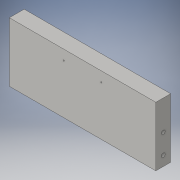
# Autodesk Inventor part: SideWall
Saved by Autodesk Inventor 2016 (Build 200138000, 138)
## iProperties
Created: 2017-01-04
Part Number: SideWall
Material: Generic
Document SubType Name: Modeling
Designer: james
Density: 1 g/cm^3
Appearance: Default
Author: james
Autodesk Inventor part; units mm, degrees
ref_plane "YZ Plane" through (0, 0, 0) normal (1, 0, 0) x (0, 1, 0)
ref_plane "XZ Plane" through (0, 0, 0) normal (0, 1, 0) x (-1, 0, 0)
ref_plane "XY Plane" through (0, 0, 0) normal (0, 0, 1) x (1, 0, 0)
sketch "Sketch1" plane through (0, 0, 0) normal (0, 1, 0) x (-1, 0, 0)
  line L0 (75.3001, 36.8452) -> (-112.6599, 36.8452)
  line L1 (-112.6599, 36.8452) -> (-112.6599, 17.7952)
  line L2 (-112.6599, 17.7952) -> (75.3001, 17.7952)
  line L3 (75.3001, 17.7952) -> (75.3001, 36.8452)
  point P0 (0, 0)
  dimension "d0" = 187.96
  dimension "d1" = 19.05
  constraints: 8 end point, 2 parallel, 1 horizontal, 1 perpendicular
  measures "d0" distance of L1.end L2.end
  measures "d1" distance of L2.end L0.start
extrude "Extrusion1" add sketch "Sketch1" along normal blind 76.2
sketch "Sketch2" plane through (112.6599, 0, 36.8452) normal (1, 0, 0) x (0, 0, -1)
  line L0 (0, 0) -> (0, 76.2) projected
  line L1 (0, 0) -> (19.05, 0) projected
  point P0 (36.8452, 0)
  point P1 (9.525, 12.7)
  point P2 (9.525, 38.1)
  dimension "d4" = 0
  dimension "d5" = 9.525
  dimension "d6" = 25.4
  dimension "d7" = 12.7
  measures "d4" horizontal distance of point (9.525, 12.7) point (9.525, 38.1)
  measures "d5" distance from line of L0 point (9.525, 38.1)
  measures "d6" distance of point (9.525, 12.7) point (9.525, 38.1)
  measures "d7" distance from line of L1 point (9.525, 12.7)
hole "Hole1" at (112.6599, 12.7, 27.3202) at (112.6599, 38.1, 27.3202) direction (-1, 0, 0) diameter 4.9149 end through all
sketch "Sketch4" plane through (112.6599, 0, 17.7952) normal (0, 0, -1) x (-1, 0, 0)
  line L0 (19.05, 57.15) -> (168.91, 57.15)
  line L1 (168.91, 57.15) -> (168.91, 12.7)
  line L2 (168.91, 12.7) -> (19.05, 12.7)
  line L3 (19.05, 12.7) -> (19.05, 57.15)
  line L4 (0, 76.2) -> (187.96, 76.2) projected
  line L5 (0, 0) -> (187.96, 0) projected
  point P0 (112.6599, 0)
  dimension "d21" = 19.05
  dimension "d22" = 12.7
  dimension "d23" = 19.05
  dimension "d24" = 19.05
  constraints: 8 end point, 2 parallel, 1 horizontal, 1 perpendicular
  measures "d21" distance between parallel lines of L0 L4
  measures "d22" distance between parallel lines of L2 L5
  measures "d23" horizontal distance of L5.end L1.end
  measures "d24" horizontal distance of L5.start L2.end
extrude "Extrusion3" cut sketch "Sketch4" against normal blind 5.08
sketch "Sketch5" plane through (112.6599, 0, 17.7952) normal (0, 0, -1) x (-1, 0, 0)
  line L0 (187.96, 0) -> (187.96, 76.2) projected
  line L1 (0, 0) -> (0, 76.2) projected
  line L2 (0, 76.2) -> (187.96, 76.2) projected
  point P0 (112.6599, 0)
  point P1 (69.85, 63.5)
  point P2 (118.11, 63.5)
  dimension "d27" = 48.26
  dimension "d28" = 69.85
  dimension "d30" = 12.7
  dimension "d31" = 12.7
  dimension "d32" = 69.85
  measures "d27" distance of point (69.85, 63.5) point (118.11, 63.5)
  measures "d28" distance from line of L0 point (118.11, 63.5)
  measures "d30" distance from line of point (69.85, 63.5) L2
  measures "d31" distance from line of point (118.11, 63.5) L2
  measures "d32" horizontal distance of point (69.85, 63.5) L1.end
hole "Hole2" at (42.8099, 63.5, 17.7952) at (-5.4501, 63.5, 17.7952) direction (0, 0, 1) diameter 1.524 end through all
sketch "Sketch6" plane through (112.6599, 0, 22.8752) normal (0, 0, -1) x (-1, 0, 0)
  line L0 (25.8304, 53.7302) -> (132.9321, 53.7302) construction
  line L1 (132.9321, 53.7302) -> (132.9321, 26.2821) construction
  line L2 (132.9321, 26.2821) -> (25.8304, 26.2821) construction
  line L3 (25.8304, 26.2821) -> (25.8304, 53.7302) construction
  line L4 (34.7951, 51.1546) -> (34.7951, 41.0658)
  line L5 (34.7951, 41.0658) -> (36.5312, 41.0658)
  spline S0 degree 2 poles (36.5312, 41.0658) (37.4988, 41.0658) (38.2957, 40.3543) (38.2957, 39.7709) knots 0 0 0 1 2 2 2
  spline S1 degree 2 poles (38.2957, 39.7709) (38.2957, 39.1875) (37.4988, 38.4902) (36.5312, 38.4902) knots 0 0 0 1 2 2 2
  line L6 (36.5312, 38.4902) -> (30.4978, 38.4902)
  spline S2 degree 2 poles (30.4978, 38.4902) (29.5302, 38.4902) (28.7333, 39.2017) (28.7333, 39.7851) knots 0 0 0 1 2 2 2
  spline S3 degree 2 poles (28.7333, 39.7851) (28.7333, 40.3685) (29.5302, 41.0658) (30.4978, 41.0658) knots 0 0 0 1 2 2 2
  line L7 (30.4978, 41.0658) -> (32.2196, 41.0658)
  line L8 (32.2196, 41.0658) -> (32.2196, 51.1546)
  line L9 (32.2196, 51.1546) -> (29.4306, 51.1546)
  line L10 (29.4306, 51.1546) -> (29.4306, 48.7214)
  spline S4 degree 2 poles (29.4306, 48.7214) (29.4306, 47.7537) (28.7191, 46.9569) (28.1357, 46.9569) knots 0 0 0 1 2 2 2
  spline S5 degree 2 poles (28.1357, 46.9569) (27.5522, 46.9569) (26.855, 47.7537) (26.855, 48.7214) knots 0 0 0 1 2 2 2
  line L11 (26.855, 48.7214) -> (26.855, 53.7302)
  line L12 (26.855, 53.7302) -> (40.2024, 53.7302)
  line L13 (40.2024, 53.7302) -> (40.2024, 48.7214)
  spline S6 degree 2 poles (40.2024, 48.7214) (40.2024, 47.7537) (39.4909, 46.9569) (38.9075, 46.9569) knots 0 0 0 1 2 2 2
  spline S7 degree 2 poles (38.9075, 46.9569) (38.3241, 46.9569) (37.6269, 47.7537) (37.6269, 48.7214) knots 0 0 0 1 2 2 2
  line L14 (37.6269, 48.7214) -> (37.6269, 51.1546)
  line L15 (37.6269, 51.1546) -> (34.7951, 51.1546)
  line L16 (55.4567, 42.8872) -> (44.884, 42.8872)
  spline S8 degree 2 poles (44.884, 42.8872) (45.2824, 41.8769) (47.3315, 40.6531) (49.0818, 40.6531) knots 0 0 0 1 2 2 2
  spline S9 degree 2 poles (49.0818, 40.6531) (50.519, 40.6531) (52.8953, 41.265) knots 0 0 0 1 1 1
  spline S10 degree 2 poles (52.8953, 41.265) (53.8772, 41.5211) (54.2471, 41.5211) knots 0 0 0 1 1 1
  spline S11 degree 2 poles (54.2471, 41.5211) (54.7736, 41.5211) (55.4709, 40.7954) (55.4709, 40.2405) knots 0 0 0 1 2 2 2
  spline S12 degree 2 poles (55.4709, 40.2405) (55.4709, 39.7424) (55.1009, 39.3867) knots 0 0 0 1 1 1
  spline S13 degree 2 poles (55.1009, 39.3867) (54.5887, 38.9171) (50.6897, 38.0776) (48.8968, 38.0776) knots 0 0 0 1 2 2 2
  spline S14 degree 2 poles (48.8968, 38.0776) (45.8089, 38.0776) (42.095, 41.5638) (42.095, 44.1109) knots 0 0 0 1 2 2 2
  spline S15 degree 2 poles (42.095, 44.1109) (42.095, 46.8288) (46.1078, 50.2297) (48.726, 50.2297) knots 0 0 0 1 2 2 2
  spline S16 degree 2 poles (48.726, 50.2297) (50.2913, 50.2297) (52.9238, 49.1198) (53.5641, 48.4795) knots 0 0 0 1 2 2 2
  spline S17 degree 2 poles (53.5641, 48.4795) (54.4606, 47.5545) (55.0582, 46.1885) knots 0 0 0 1 1 1
  spline S18 degree 2 poles (55.0582, 46.1885) (55.4567, 45.2351) (55.4567, 43.9829) knots 0 0 0 1 1 1
  line L17 (55.4567, 43.9829) -> (55.4567, 42.8872)
  spline S19 degree 2 poles (52.6107, 45.4628) (52.0131, 46.5584) (50.1063, 47.6541) (48.7829, 47.6541) knots 0 0 0 1 2 2 2
  spline S20 degree 2 poles (48.7829, 47.6541) (47.4738, 47.6541) (45.5528, 46.5584) (44.9551, 45.4628) knots 0 0 0 1 2 2 2
  line L18 (44.9551, 45.4628) -> (52.6107, 45.4628)
  line L19 (66.7408, 38.4902) -> (66.7408, 39.0879)
  spline S21 degree 2 poles (66.7408, 39.0879) (65.7732, 38.5898) (63.4395, 38.0776) (62.4861, 38.0776) knots 0 0 0 1 2 2 2
  spline S22 degree 2 poles (62.4861, 38.0776) (60.4228, 38.0776) (57.833, 40.2689) (57.833, 41.5923) knots 0 0 0 1 2 2 2
  spline S23 degree 2 poles (57.833, 41.5923) (57.833, 43.2145) (61.1343, 45.975) (64.0372, 45.975) knots 0 0 0 1 2 2 2
  spline S24 degree 2 poles (64.0372, 45.975) (65.204, 45.975) (66.7408, 45.7189) knots 0 0 0 1 1 1
  line L20 (66.7408, 45.7189) -> (66.7408, 46.345)
  spline S25 degree 2 poles (66.7408, 46.345) (66.7408, 46.9284) (65.7447, 47.6541) (64.3644, 47.6541) knots 0 0 0 1 2 2 2
  spline S26 degree 2 poles (64.3644, 47.6541) (63.2118, 47.6541) (61.3904, 47.1988) knots 0 0 0 1 1 1
  spline S27 degree 2 poles (61.3904, 47.1988) (60.7216, 47.0423) (60.3374, 47.0423) knots 0 0 0 1 1 1
  spline S28 degree 2 poles (60.3374, 47.0423) (59.8252, 47.0423) (59.1137, 47.7822) (59.1137, 48.3656) knots 0 0 0 1 2 2 2
  spline S29 degree 2 poles (59.1137, 48.3656) (59.1137, 48.6929) (59.3698, 49.1625) (59.8109, 49.4471) (60.5367, 49.6463) knots 0 0 0 1 2 3 3 3
  spline S30 degree 2 poles (60.5367, 49.6463) (61.4901, 49.9167) (63.468, 50.2297) (64.2648, 50.2297) knots 0 0 0 1 2 2 2
  spline S31 degree 2 poles (64.2648, 50.2297) (66.6697, 50.2297) (69.3164, 48.1522) (69.3164, 46.3592) knots 0 0 0 1 2 2 2
  line L21 (69.3164, 46.3592) -> (69.3164, 41.0658)
  line L22 (69.3164, 41.0658) -> (69.7575, 41.0658)
  spline S32 degree 2 poles (69.7575, 41.0658) (70.7251, 41.0658) (71.522, 40.3543) (71.522, 39.7709) knots 0 0 0 1 2 2 2
  spline S33 degree 2 poles (71.522, 39.7709) (71.522, 39.1875) (70.7251, 38.4902) (69.7575, 38.4902) knots 0 0 0 1 2 2 2
  line L23 (69.7575, 38.4902) -> (66.7408, 38.4902)
  spline S34 degree 2 poles (66.7408, 43.1006) (65.204, 43.3995) (63.8949, 43.3995) knots 0 0 0 1 1 1
  spline S35 degree 2 poles (63.8949, 43.3995) (62.3296, 43.3995) (61.1912, 42.6311) knots 0 0 0 1 1 1
  spline S36 degree 2 poles (61.1912, 42.6311) (60.494, 42.1472) (60.494, 41.6492) knots 0 0 0 1 1 1
  spline S37 degree 2 poles (60.494, 41.6492) (60.494, 41.2935) (60.8355, 41.0658) knots 0 0 0 1 1 1
  spline S38 degree 2 poles (60.8355, 41.0658) (61.4616, 40.6531) (62.5573, 40.6531) knots 0 0 0 1 1 1
  spline S39 degree 2 poles (62.5573, 40.6531) (63.4822, 40.6531) (65.8301, 41.3788) (66.7408, 42.0049) knots 0 0 0 1 2 2 2
  line L24 (66.7408, 42.0049) -> (66.7408, 43.1006)
  line L25 (75.8905, 49.9024) -> (75.8905, 49.1767)
  spline S40 degree 2 poles (75.8905, 49.1767) (76.5166, 49.7886) (77.5411, 50.2439) (78.2099, 50.2439) knots 0 0 0 1 2 2 2
  spline S41 degree 2 poles (78.2099, 50.2439) (78.7649, 50.2439) (79.8748, 49.689) (80.4013, 49.1483) knots 0 0 0 1 2 2 2
  spline S42 degree 2 poles (80.4013, 49.1483) (81.0701, 49.689) (82.4362, 50.2297) (83.1619, 50.2297) knots 0 0 0 1 2 2 2
  spline S43 degree 2 poles (83.1619, 50.2297) (84.5848, 50.2297) (85.4813, 49.4613) knots 0 0 0 1 1 1
  spline S44 degree 2 poles (85.4813, 49.4613) (86.6624, 48.4652) (86.6624, 46.8288) knots 0 0 0 1 1 1
  line L26 (86.6624, 46.8288) -> (86.6624, 41.0658)
  spline S45 degree 2 poles (86.6624, 41.0658) (87.63, 41.0658) (88.4269, 40.3543) (88.4269, 39.7709) knots 0 0 0 1 2 2 2
  spline S46 degree 2 poles (88.4269, 39.7709) (88.4269, 39.1875) (87.63, 38.4902) (86.6624, 38.4902) knots 0 0 0 1 2 2 2
  line L27 (86.6624, 38.4902) -> (84.0868, 38.4902)
  line L28 (84.0868, 38.4902) -> (84.0868, 46.6154)
  spline S47 degree 2 poles (84.0868, 46.6154) (84.0868, 47.1988) (83.6599, 47.6541) (83.2188, 47.6541) knots 0 0 0 1 2 2 2
  spline S48 degree 2 poles (83.2188, 47.6541) (82.7919, 47.6541) (82.4219, 47.4265) knots 0 0 0 1 1 1
  spline S49 degree 2 poles (82.4219, 47.4265) (81.9666, 47.1134) (81.2978, 46.2596) knots 0 0 0 1 1 1
  line L29 (81.2978, 46.2596) -> (81.2978, 41.0658)
  spline S50 degree 2 poles (81.2978, 41.0658) (82.2654, 41.0658) (83.0623, 40.3543) (83.0623, 39.7709) knots 0 0 0 1 2 2 2
  spline S51 degree 2 poles (83.0623, 39.7709) (83.0623, 39.1875) (82.2654, 38.4902) (81.2978, 38.4902) knots 0 0 0 1 2 2 2
  line L30 (81.2978, 38.4902) -> (78.7222, 38.4902)
  line L31 (78.7222, 38.4902) -> (78.7222, 46.6296)
  spline S52 degree 2 poles (78.7222, 46.6296) (78.7222, 47.1988) (78.2811, 47.6684) (77.84, 47.6684) knots 0 0 0 1 2 2 2
  spline S53 degree 2 poles (77.84, 47.6684) (77.3846, 47.6684) (76.5024, 47.0992) (75.8905, 46.2596) knots 0 0 0 1 2 2 2
  line L32 (75.8905, 46.2596) -> (75.8905, 41.0658)
  spline S54 degree 2 poles (75.8905, 41.0658) (76.8581, 41.0658) (77.655, 40.3543) (77.655, 39.7709) knots 0 0 0 1 2 2 2
  spline S55 degree 2 poles (77.655, 39.7709) (77.655, 39.1875) (76.8581, 38.4902) (75.8905, 38.4902) knots 0 0 0 1 2 2 2
  line L33 (75.8905, 38.4902) -> (73.3149, 38.4902)
  spline S56 degree 2 poles (73.3149, 38.4902) (72.3473, 38.4902) (71.5504, 39.2017) (71.5504, 39.7851) knots 0 0 0 1 2 2 2
  spline S57 degree 2 poles (71.5504, 39.7851) (71.5504, 40.3685) (72.3473, 41.0658) (73.3149, 41.0658) knots 0 0 0 1 2 2 2
  line L34 (73.3149, 41.0658) -> (73.3149, 47.3269)
  spline S58 degree 2 poles (73.3149, 47.3269) (72.3473, 47.3269) (71.5504, 48.0383) (71.5504, 48.6218) knots 0 0 0 1 2 2 2
  spline S59 degree 2 poles (71.5504, 48.6218) (71.5504, 49.2052) (72.3473, 49.9024) (73.3149, 49.9024) knots 0 0 0 1 2 2 2
  line L35 (73.3149, 49.9024) -> (75.8905, 49.9024)
  point P0 (112.6599, 0)
  constraints: 2 other
extrude "Extrusion4" add sketch "Sketch6" along normal blind 2.54
sketch "Sketch7" plane through (112.6599, 0, 22.8752) normal (0, 0, -1) x (-1, 0, 0)
  line L0 (44.6427, 45.8411) -> (161.4517, 31.4988) construction
  line L1 (161.4517, 31.4988) -> (158.1503, 4.6114) construction
  line L2 (158.1503, 4.6114) -> (41.3413, 18.9537) construction
  line L3 (41.3413, 18.9537) -> (44.6427, 45.8411) construction
  line L4 (48.3943, 34.8288) -> (47.9989, 31.6086)
  line L5 (47.9989, 31.6086) -> (48.917, 31.4959)
  spline S0 degree 2 poles (48.917, 31.4959) (49.8774, 31.3779) (50.5816, 30.5747) (50.5105, 29.9956) knots 0 0 0 1 2 2 2
  spline S1 degree 2 poles (50.5105, 29.9956) (50.4394, 29.4165) (49.5635, 28.8216) (48.6031, 28.9395) knots 0 0 0 1 2 2 2
  line L6 (48.6031, 28.9395) -> (44.7332, 29.4147)
  spline S2 degree 2 poles (44.7332, 29.4147) (43.7728, 29.5326) (43.0686, 30.3359) (43.1397, 30.9149) knots 0 0 0 1 2 2 2
  spline S3 degree 2 poles (43.1397, 30.9149) (43.2108, 31.494) (44.0867, 32.089) (45.0471, 31.971) knots 0 0 0 1 2 2 2
  line L7 (45.0471, 31.971) -> (45.4426, 31.9225)
  line L8 (45.4426, 31.9225) -> (46.6721, 41.9361)
  line L9 (46.6721, 41.9361) -> (46.2766, 41.9847)
  spline S4 degree 2 poles (46.2766, 41.9847) (45.3162, 42.1026) (44.612, 42.9059) (44.6831, 43.485) knots 0 0 0 1 2 2 2
  spline S5 degree 2 poles (44.6831, 43.485) (44.7525, 44.0499) (45.6301, 44.659) (46.5905, 44.5411) knots 0 0 0 1 2 2 2
  line L10 (46.5905, 44.5411) -> (52.3795, 43.8159)
  spline S6 degree 2 poles (52.3795, 43.8159) (55.0771, 43.4847) (57.7277, 40.4353) (57.4918, 38.5145) knots 0 0 0 1 2 2 2
  spline S7 degree 2 poles (57.4918, 38.5145) (57.3462, 37.3281) (55.7069, 35.5366) (54.2009, 34.9473) knots 0 0 0 1 2 2 2
  spline S8 degree 2 poles (54.2009, 34.9473) (54.9333, 34.1406) (55.7144, 32.9121) knots 0 0 0 1 1 1
  spline S9 degree 2 poles (55.7144, 32.9121) (56.2067, 32.1348) (56.9957, 30.5039) knots 0 0 0 1 1 1
  spline S10 degree 2 poles (56.9957, 30.5039) (57.9561, 30.386) (58.2091, 30.1112) knots 0 0 0 1 1 1
  spline S11 degree 2 poles (58.2091, 30.1112) (58.6603, 29.5827) (58.5892, 29.0036) knots 0 0 0 1 1 1
  spline S12 degree 2 poles (58.5892, 29.0036) (58.5181, 28.4246) (57.6422, 27.8296) (56.6818, 27.9475) knots 0 0 0 1 2 2 2
  line L11 (56.6818, 27.9475) -> (55.3683, 28.1088)
  spline S13 degree 2 poles (55.3683, 28.1088) (52.8507, 33.2924) (50.9225, 34.5184) knots 0 0 0 1 1 1
  line L12 (50.9225, 34.5184) -> (48.3943, 34.8288)
  line L13 (48.7082, 37.3852) -> (50.6996, 37.1406)
  spline S14 degree 2 poles (50.6996, 37.1406) (51.8154, 37.0036) (52.7327, 37.2351) knots 0 0 0 1 1 1
  spline S15 degree 2 poles (52.7327, 37.2351) (53.9605, 37.5431) (54.8869, 38.4329) (54.9476, 38.9272) knots 0 0 0 1 2 2 2
  spline S16 degree 2 poles (54.9476, 38.9272) (55.036, 39.6475) (53.6474, 41.0653) (52.1503, 41.2491) knots 0 0 0 1 2 2 2
  line L14 (52.1503, 41.2491) -> (49.2285, 41.6222)
  line L15 (49.2285, 41.6222) -> (48.7082, 37.3852)
  line L16 (72.5983, 30.4232) -> (62.1044, 31.7117)
  spline S17 degree 2 poles (62.1044, 31.7117) (62.3768, 30.6604) (64.2614, 29.196) (65.9986, 28.9827) knots 0 0 0 1 2 2 2
  spline S18 degree 2 poles (65.9986, 28.9827) (67.4251, 28.8076) (69.8583, 29.1253) knots 0 0 0 1 1 1
  spline S19 degree 2 poles (69.8583, 29.1253) (70.8641, 29.2599) (71.2313, 29.2148) knots 0 0 0 1 1 1
  spline S20 degree 2 poles (71.2313, 29.2148) (71.7539, 29.1506) (72.3575, 28.3453) (72.2899, 27.7945) knots 0 0 0 1 2 2 2
  spline S21 degree 2 poles (72.2899, 27.7945) (72.2292, 27.3002) (71.8186, 26.9922) knots 0 0 0 1 1 1
  spline S22 degree 2 poles (71.8186, 26.9922) (71.2529, 26.5885) (67.2807, 26.2304) (65.5012, 26.4489) knots 0 0 0 1 2 2 2
  spline S23 degree 2 poles (65.5012, 26.4489) (62.4363, 26.8252) (59.1749, 30.7381) (59.4853, 33.2663) knots 0 0 0 1 2 2 2
  spline S24 degree 2 poles (59.4853, 33.2663) (59.8166, 35.9639) (64.2139, 38.8504) (66.8126, 38.5313) knots 0 0 0 1 2 2 2
  spline S25 degree 2 poles (66.8126, 38.5313) (68.3662, 38.3405) (70.8439, 36.9181) (71.4014, 36.2045) knots 0 0 0 1 2 2 2
  spline S26 degree 2 poles (71.4014, 36.2045) (72.1784, 35.1772) (72.6052, 33.7485) knots 0 0 0 1 1 1
  spline S27 degree 2 poles (72.6052, 33.7485) (72.8844, 32.7536) (72.7318, 31.5108) knots 0 0 0 1 1 1
  line L17 (72.7318, 31.5108) -> (72.5983, 30.4232)
  spline S28 degree 2 poles (70.0875, 33.3265) (69.6278, 34.4868) (67.8688, 35.8067) (66.5553, 35.968) knots 0 0 0 1 2 2 2
  spline S29 degree 2 poles (66.5553, 35.968) (65.2559, 36.1275) (63.2157, 35.2741) (62.4889, 34.2594) knots 0 0 0 1 2 2 2
  line L18 (62.4889, 34.2594) -> (70.0875, 33.3265)
  line L19 (88.8072, 40.4184) -> (87.1355, 26.8032)
  line L20 (87.1355, 26.8032) -> (87.5733, 26.7495)
  spline S30 degree 2 poles (87.5733, 26.7495) (88.5337, 26.6315) (89.238, 25.8282) (89.1669, 25.2492) knots 0 0 0 1 2 2 2
  spline S31 degree 2 poles (89.1669, 25.2492) (89.0958, 24.6701) (88.2199, 24.0752) (87.2595, 24.1931) knots 0 0 0 1 2 2 2
  line L21 (87.2595, 24.1931) -> (84.2652, 24.5607)
  line L22 (84.2652, 24.5607) -> (84.3416, 25.1822)
  spline S32 degree 2 poles (84.3416, 25.1822) (83.4035, 24.7812) (81.4326, 24.4928) (80.4157, 24.6176) knots 0 0 0 1 2 2 2
  spline S33 degree 2 poles (80.4157, 24.6176) (77.5486, 24.9697) (74.4411, 28.7347) (74.7446, 31.2063) knots 0 0 0 1 2 2 2
  spline S34 degree 2 poles (74.7446, 31.2063) (75.0637, 33.805) (79.1991, 37.0104) (81.8543, 36.6844) knots 0 0 0 1 2 2 2
  spline S35 degree 2 poles (81.8543, 36.6844) (82.843, 36.563) (84.6892, 35.7199) (85.5451, 34.984) knots 0 0 0 1 2 2 2
  line L23 (85.5451, 34.984) -> (85.937, 38.1759)
  line L24 (85.937, 38.1759) -> (85.4992, 38.2297)
  spline S36 degree 2 poles (85.4992, 38.2297) (84.5387, 38.3476) (83.8328, 39.1368) (83.9039, 39.7158) knots 0 0 0 1 2 2 2
  spline S37 degree 2 poles (83.9039, 39.7158) (83.975, 40.2949) (84.8526, 40.904) (85.813, 40.786) knots 0 0 0 1 2 2 2
  line L25 (85.813, 40.786) -> (88.8072, 40.4184)
  spline S38 degree 2 poles (84.919, 29.8853) (85.1133, 31.4672) (83.1646, 33.9286) (81.5687, 34.1246) knots 0 0 0 1 2 2 2
  spline S39 degree 2 poles (81.5687, 34.1246) (79.9727, 34.3205) (77.4865, 32.4036) (77.2957, 30.85) knots 0 0 0 1 2 2 2
  spline S40 degree 2 poles (77.2957, 30.85) (77.1241, 29.4518) (78.8935, 27.3995) (80.7155, 27.1757) knots 0 0 0 1 2 2 2
  spline S41 degree 2 poles (80.7155, 27.1757) (82.5092, 26.9555) (84.7508, 28.5153) (84.919, 29.8853) knots 0 0 0 1 2 2 2
  line L26 (98.5866, 22.8023) -> (98.6594, 23.3955)
  spline S42 degree 2 poles (98.6594, 23.3955) (97.6383, 23.0191) (95.2596, 22.795) (94.3134, 22.9112) knots 0 0 0 1 2 2 2
  spline S43 degree 2 poles (94.3134, 22.9112) (92.2654, 23.1627) (89.962, 25.6533) (90.1233, 26.9668) knots 0 0 0 1 2 2 2
  spline S44 degree 2 poles (90.1233, 26.9668) (90.321, 28.5769) (93.9341, 30.9146) (96.8153, 30.5608) knots 0 0 0 1 2 2 2
  spline S45 degree 2 poles (96.8153, 30.5608) (97.9734, 30.4186) (99.4676, 29.9771) knots 0 0 0 1 1 1
  line L27 (99.4676, 29.9771) -> (99.5439, 30.5985)
  spline S46 degree 2 poles (99.5439, 30.5985) (99.615, 31.1776) (98.7148, 32.0193) (97.3448, 32.1875) knots 0 0 0 1 2 2 2
  spline S47 degree 2 poles (97.3448, 32.1875) (96.2007, 32.328) (94.3374, 32.098) knots 0 0 0 1 1 1
  spline S48 degree 2 poles (94.3374, 32.098) (93.6545, 32.0241) (93.2732, 32.071) knots 0 0 0 1 1 1
  spline S49 degree 2 poles (93.2732, 32.071) (92.7648, 32.1334) (92.1488, 32.9545) (92.2199, 33.5336) knots 0 0 0 1 2 2 2
  spline S50 degree 2 poles (92.2199, 33.5336) (92.2597, 33.8584) (92.5712, 34.2933) (93.0437, 34.522) (93.7883, 34.6313) knots 0 0 0 1 2 3 3 3
  spline S51 degree 2 poles (93.7883, 34.6313) (94.7675, 34.7835) (96.7689, 34.8531) (97.5598, 34.756) knots 0 0 0 1 2 2 2
  spline S52 degree 2 poles (97.5598, 34.756) (99.9467, 34.463) (102.3205, 32.0783) (102.102, 30.2988) knots 0 0 0 1 2 2 2
  line L28 (102.102, 30.2988) -> (101.4569, 25.0448)
  line L29 (101.4569, 25.0448) -> (101.8947, 24.991)
  spline S53 degree 2 poles (101.8947, 24.991) (102.8551, 24.8731) (103.5593, 24.0698) (103.4882, 23.4907) knots 0 0 0 1 2 2 2
  spline S54 degree 2 poles (103.4882, 23.4907) (103.4171, 22.9117) (102.5412, 22.3167) (101.5808, 22.4346) knots 0 0 0 1 2 2 2
  line L30 (101.5808, 22.4346) -> (98.5866, 22.8023)
  spline S55 degree 2 poles (99.1485, 27.3783) (97.6595, 27.8622) (96.3602, 28.0218) knots 0 0 0 1 1 1
  spline S56 degree 2 poles (96.3602, 28.0218) (94.8066, 28.2125) (93.583, 27.5886) knots 0 0 0 1 1 1
  spline S57 degree 2 poles (93.583, 27.5886) (92.832, 27.1934) (92.7713, 26.699) knots 0 0 0 1 1 1
  spline S58 degree 2 poles (92.7713, 26.699) (92.728, 26.3459) (93.0392, 26.0783) knots 0 0 0 1 1 1
  spline S59 degree 2 poles (93.0392, 26.0783) (93.6103, 25.5925) (94.6979, 25.4589) knots 0 0 0 1 1 1
  spline S60 degree 2 poles (94.6979, 25.4589) (95.6159, 25.3462) (98.0347, 25.7804) (99.0149, 26.2908) knots 0 0 0 1 2 2 2
  line L31 (99.0149, 26.2908) -> (99.1485, 27.3783)
  spline S61 degree 2 poles (116.9374, 31.5596) (117.4449, 31.956) (117.9392, 31.8953) knots 0 0 0 1 1 1
  spline S62 degree 2 poles (117.9392, 31.8953) (118.49, 31.8277) (119.0991, 30.9501) (118.9881, 30.0462) knots 0 0 0 1 2 2 2
  line L32 (118.9881, 30.0462) -> (118.7852, 28.3937)
  spline S63 degree 2 poles (118.7852, 28.3937) (118.6725, 27.4757) (117.8709, 26.7856) (117.2918, 26.8567) knots 0 0 0 1 2 2 2
  spline S64 degree 2 poles (117.2918, 26.8567) (116.7693, 26.9208) (116.4385, 27.2625) knots 0 0 0 1 1 1
  spline S65 degree 2 poles (116.4385, 27.2625) (116.212, 27.5197) (116.0853, 28.9402) (115.5479, 29.3503) knots 0 0 0 1 2 2 2
  spline S66 degree 2 poles (115.5479, 29.3503) (114.618, 30.0666) (113.0361, 30.2609) knots 0 0 0 1 1 1
  spline S67 degree 2 poles (113.0361, 30.2609) (111.2283, 30.4828) (108.7931, 28.6313) (108.5954, 27.0212) knots 0 0 0 1 2 2 2
  spline S68 degree 2 poles (108.5954, 27.0212) (108.4116, 25.5241) (110.2903, 23.5444) (112.7196, 23.2461) knots 0 0 0 1 2 2 2
  spline S69 degree 2 poles (112.7196, 23.2461) (114.3156, 23.0502) (115.3724, 23.2502) knots 0 0 0 1 1 1
  spline S70 degree 2 poles (115.3724, 23.2502) (115.9898, 23.375) (117.1811, 24.2037) (117.619, 24.1499) knots 0 0 0 1 2 2 2
  spline S71 degree 2 poles (117.619, 24.1499) (118.1416, 24.0857) (118.8088, 23.2153) (118.7447, 22.6927) knots 0 0 0 1 2 2 2
  spline S72 degree 2 poles (118.7447, 22.6927) (118.6406, 21.8453) (117.3889, 21.2248) knots 0 0 0 1 1 1
  spline S73 degree 2 poles (117.3889, 21.2248) (115.527, 20.3065) (112.208, 20.714) knots 0 0 0 1 1 1
  spline S74 degree 2 poles (112.208, 20.714) (109.2279, 21.0799) (107.7263, 22.5116) knots 0 0 0 1 1 1
  spline S75 degree 2 poles (107.7263, 22.5116) (105.6835, 24.4398) (106.0373, 27.321) knots 0 0 0 1 1 1
  spline S76 degree 2 poles (106.0373, 27.321) (106.372, 30.0469) (110.4547, 33.1727) (113.3782, 32.8138) knots 0 0 0 1 2 2 2
  spline S77 degree 2 poles (113.3782, 32.8138) (114.4375, 32.6837) (116.2109, 32.0645) (116.9374, 31.5596) knots 0 0 0 1 2 2 2
  line L33 (127.3882, 28.1689) -> (126.7587, 23.042)
  spline S78 degree 2 poles (126.7587, 23.042) (126.6581, 22.2229) (126.9641, 21.9129) knots 0 0 0 1 1 1
  spline S79 degree 2 poles (126.9641, 21.9129) (127.4364, 21.4391) (128.7782, 21.2744) knots 0 0 0 1 1 1
  spline S80 degree 2 poles (128.7782, 21.2744) (130.7413, 21.0333) (132.4961, 21.6637) knots 0 0 0 1 1 1
  spline S81 degree 2 poles (132.4961, 21.6637) (133.1716, 21.9105) (133.5388, 21.8655) knots 0 0 0 1 1 1
  spline S82 degree 2 poles (133.5388, 21.8655) (134.0331, 21.8048) (134.6756, 20.966) (134.6097, 20.4293) knots 0 0 0 1 2 2 2
  spline S83 degree 2 poles (134.6097, 20.4293) (134.549, 19.935) (134.1085, 19.6163) knots 0 0 0 1 1 1
  spline S84 degree 2 poles (134.1085, 19.6163) (133.4301, 19.1118) (129.693, 18.5671) (128.4643, 18.718) knots 0 0 0 1 2 2 2
  spline S85 degree 2 poles (128.4643, 18.718) (126.0915, 19.0093) (123.9578, 21.3645) (124.1416, 22.8616) knots 0 0 0 1 2 2 2
  line L34 (124.1416, 22.8616) -> (124.8318, 28.4828)
  line L35 (124.8318, 28.4828) -> (123.9138, 28.5955)
  spline S86 degree 2 poles (123.9138, 28.5955) (122.9958, 28.7082) (122.2915, 29.5115) (122.3626, 30.0906) knots 0 0 0 1 2 2 2
  spline S87 degree 2 poles (122.3626, 30.0906) (122.432, 30.6555) (123.3096, 31.2646) (124.2277, 31.1519) knots 0 0 0 1 2 2 2
  line L36 (124.2277, 31.1519) -> (125.1457, 31.0392)
  line L37 (125.1457, 31.0392) -> (125.4284, 33.3413)
  spline S88 degree 2 poles (125.4284, 33.3413) (125.5411, 34.2593) (126.3444, 34.9636) (126.9235, 34.8925) knots 0 0 0 1 2 2 2
  spline S89 degree 2 poles (126.9235, 34.8925) (127.4884, 34.8231) (128.0975, 33.9455) (127.9848, 33.0274) knots 0 0 0 1 2 2 2
  line L38 (127.9848, 33.0274) -> (127.7021, 30.7253)
  line L39 (127.7021, 30.7253) -> (132.4194, 30.1461)
  spline S90 degree 2 poles (132.4194, 30.1461) (133.3374, 30.0333) (134.0416, 29.23) (133.9705, 28.651) knots 0 0 0 1 2 2 2
  spline S91 degree 2 poles (133.9705, 28.651) (133.9012, 28.086) (133.0235, 27.477) (132.1055, 27.5897) knots 0 0 0 1 2 2 2
  line L40 (132.1055, 27.5897) -> (127.3882, 28.1689)
  line L41 (149.219, 21.0154) -> (138.7251, 22.3039)
  spline S92 degree 2 poles (138.7251, 22.3039) (138.9974, 21.2526) (140.8821, 19.7882) (142.6193, 19.5749) knots 0 0 0 1 2 2 2
  spline S93 degree 2 poles (142.6193, 19.5749) (144.0458, 19.3998) (146.479, 19.7175) knots 0 0 0 1 1 1
  spline S94 degree 2 poles (146.479, 19.7175) (147.4848, 19.852) (147.852, 19.8069) knots 0 0 0 1 1 1
  spline S95 degree 2 poles (147.852, 19.8069) (148.3746, 19.7428) (148.9782, 18.9375) (148.9105, 18.3867) knots 0 0 0 1 2 2 2
  spline S96 degree 2 poles (148.9105, 18.3867) (148.8498, 17.8924) (148.4393, 17.5844) knots 0 0 0 1 1 1
  spline S97 degree 2 poles (148.4393, 17.5844) (147.8736, 17.1807) (143.9014, 16.8226) (142.1218, 17.0411) knots 0 0 0 1 2 2 2
  spline S98 degree 2 poles (142.1218, 17.0411) (139.057, 17.4174) (135.7956, 21.3303) (136.106, 23.8584) knots 0 0 0 1 2 2 2
  spline S99 degree 2 poles (136.106, 23.8584) (136.4372, 26.556) (140.8346, 29.4425) (143.4333, 29.1235) knots 0 0 0 1 2 2 2
  spline S100 degree 2 poles (143.4333, 29.1235) (144.9869, 28.9327) (147.4645, 27.5102) (148.022, 26.7966) knots 0 0 0 1 2 2 2
  spline S101 degree 2 poles (148.022, 26.7966) (148.7991, 25.7694) (149.2258, 24.3406) knots 0 0 0 1 1 1
  spline S102 degree 2 poles (149.2258, 24.3406) (149.5051, 23.3458) (149.3525, 22.1029) knots 0 0 0 1 1 1
  line L42 (149.3525, 22.1029) -> (149.219, 21.0154)
  spline S103 degree 2 poles (146.7081, 23.9186) (146.2485, 25.079) (144.4894, 26.3989) (143.1759, 26.5601) knots 0 0 0 1 2 2 2
  spline S104 degree 2 poles (143.1759, 26.5601) (141.8766, 26.7197) (139.8363, 25.8663) (139.1096, 24.8516) knots 0 0 0 1 2 2 2
  line L43 (139.1096, 24.8516) -> (146.7081, 23.9186)
  line L44 (165.4279, 31.0106) -> (163.7562, 17.3954)
  line L45 (163.7562, 17.3954) -> (164.194, 17.3416)
  spline S105 degree 2 poles (164.194, 17.3416) (165.1544, 17.2237) (165.8586, 16.4204) (165.7875, 15.8413) knots 0 0 0 1 2 2 2
  spline S106 degree 2 poles (165.7875, 15.8413) (165.7164, 15.2623) (164.8405, 14.6673) (163.8801, 14.7853) knots 0 0 0 1 2 2 2
  line L46 (163.8801, 14.7853) -> (160.8859, 15.1529)
  line L47 (160.8859, 15.1529) -> (160.9622, 15.7743)
  spline S107 degree 2 poles (160.9622, 15.7743) (160.0241, 15.3734) (158.0533, 15.0849) (157.0364, 15.2098) knots 0 0 0 1 2 2 2
  spline S108 degree 2 poles (157.0364, 15.2098) (154.1693, 15.5618) (151.0618, 19.3268) (151.3652, 21.7985) knots 0 0 0 1 2 2 2
  spline S109 degree 2 poles (151.3652, 21.7985) (151.6843, 24.3972) (155.8197, 27.6026) (158.475, 27.2766) knots 0 0 0 1 2 2 2
  spline S110 degree 2 poles (158.475, 27.2766) (159.4636, 27.1552) (161.3099, 26.312) (162.1657, 25.5761) knots 0 0 0 1 2 2 2
  line L48 (162.1657, 25.5761) -> (162.5577, 28.7681)
  line L49 (162.5577, 28.7681) -> (162.1198, 28.8218)
  spline S111 degree 2 poles (162.1198, 28.8218) (161.1594, 28.9398) (160.4535, 29.7289) (160.5246, 30.308) knots 0 0 0 1 2 2 2
  spline S112 degree 2 poles (160.5246, 30.308) (160.5957, 30.8871) (161.4733, 31.4961) (162.4337, 31.3782) knots 0 0 0 1 2 2 2
  line L50 (162.4337, 31.3782) -> (165.4279, 31.0106)
  spline S113 degree 2 poles (161.5397, 20.4775) (161.7339, 22.0593) (159.7853, 24.5208) (158.1893, 24.7167) knots 0 0 0 1 2 2 2
  spline S114 degree 2 poles (158.1893, 24.7167) (156.5934, 24.9127) (154.1072, 22.9958) (153.9164, 21.4422) knots 0 0 0 1 2 2 2
  spline S115 degree 2 poles (153.9164, 21.4422) (153.7447, 20.044) (155.5142, 17.9916) (157.3361, 17.7679) knots 0 0 0 1 2 2 2
  spline S116 degree 2 poles (157.3361, 17.7679) (159.1298, 17.5477) (161.3715, 19.1075) (161.5397, 20.4775) knots 0 0 0 1 2 2 2
  point P0 (112.6599, 0)
  constraints: 2 other
extrude "Extrusion5" add sketch "Sketch7" along normal blind 3.048
sketch "Sketch8" plane through (0, 0, 0) normal (0, -1, 0) x (1, 0, 0)
  line L0 (-75.3001, 17.7952) -> (-75.3001, 36.8452) projected
  line L1 (-75.3001, 36.8452) -> (112.6599, 36.8452) projected
  point P0 (0, 0)
  point P1 (70.7499, 30.4952)
  point P2 (19.9499, 27.3202)
  point P3 (-30.8501, 27.3202)
  dimension "d44" = 50.8
  dimension "d45" = 44.45
  dimension "d46" = 9.525
  dimension "d47" = 9.525
  dimension "d48" = 6.35
  dimension "d49" = 50.8
  measures "d44" distance of point (19.95, 27.32) point (-30.85, 27.32)
  measures "d45" distance from line of L0 point (-30.85, 27.32)
  measures "d46" distance from line of L1 point (-30.85, 27.32)
  measures "d47" distance from line of L1 point (19.95, 27.32)
  measures "d48" distance from line of L1 point (70.75, 30.495)
  measures "d49" horizontal distance of point (19.95, 27.32) point (70.75, 30.495)
hole "Hole3" at (70.7499, 0, 30.4952) at (19.9499, 0, 27.3202) at (-30.8501, 0, 27.3202) direction (0, 1, 0) diameter 4.9149 depth 31.75 tip angle 118
body "Solid1"
